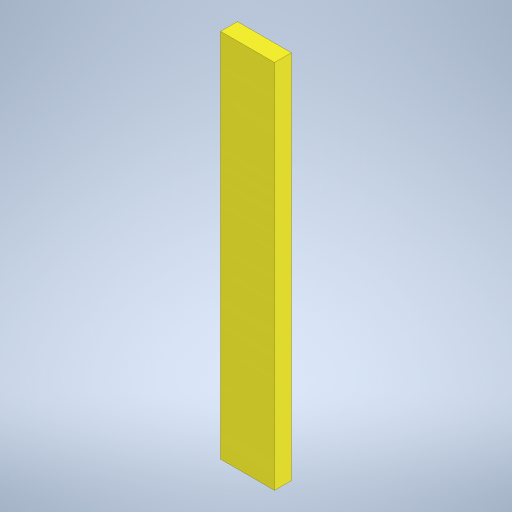
# Autodesk Inventor part: Side Plate
Saved by Autodesk Inventor 2024 (Build 280153000, 153)
## iProperties
Created: 2023-10-03
Part Number: Side Plate
Material: Generic
Document SubType Name: Modeling
Designer: flynf
Density: 1 g/cm^3
Appearance: Canary
Author: flynf
Autodesk Inventor part; units mm, degrees
ref_plane "YZ Plane" through (0, 0, 0) normal (1, 0, 0) x (0, 1, 0)
ref_plane "XZ Plane" through (0, 0, 0) normal (0, 1, 0) x (-1, 0, 0)
ref_plane "XY Plane" through (0, 0, 0) normal (0, 0, 1) x (1, 0, 0)
sketch "Sketch1" plane through (0, 0, 0) normal (0, 0, 1) x (1, 0, 0)
  line L0 (0, 0) -> (40.64, 0)
  line L1 (40.64, 0) -> (40.64, 279.4)
  line L2 (40.64, 279.4) -> (0, 279.4)
  line L3 (0, 279.4) -> (0, 0)
  constraints: 8 end point, 2 parallel, 1 horizontal, 1 perpendicular
extrude "Extrusion1" add sketch "Sketch1" along normal blind 12.7
body "Solid1"
